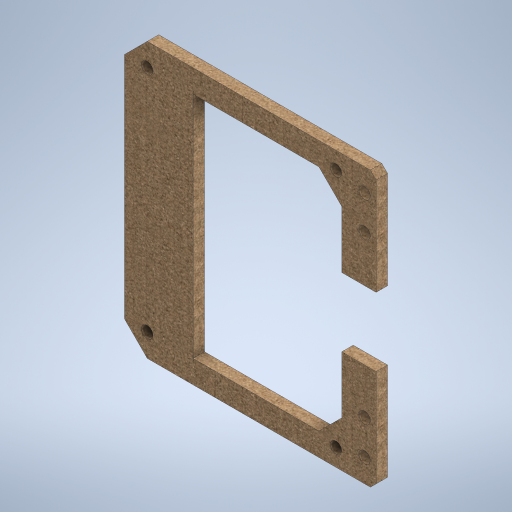
# Autodesk Inventor part: MarcoV2
Saved by Autodesk Inventor 2023.1 (Build 271208000, 208)
## iProperties
Created: 2022-10-30
Part Number: MarcoV2
Material: MDF Medium Density Fiberboard
Document SubType Name: Modeling
Designer: Daniel Peña
Density: 0.8 g/cm^3
Appearance: Cardboard - Corrugated
Author: Daniel Peña
Autodesk Inventor part; units mm, degrees
ref_plane "YZ Plane" through (0, 0, 0) normal (1, 0, 0) x (0, 1, 0)
ref_plane "XZ Plane" through (0, 0, 0) normal (0, 1, 0) x (-1, 0, 0)
ref_plane "XY Plane" through (0, 0, 0) normal (0, 0, 1) x (1, 0, 0)
sketch "Sketch1" plane through (0, 0, 0) normal (0, 0, 1) x (1, 0, 0)
  line L0 (-175, -7.5) -> (-230, -7.5)
  line L1 (-250, 2.5) -> (-152.5, 2.5)
  line L2 (-82.5, -57.5) -> (-255, -57.5)
  line L3 (-150, -42.5) -> (-165, -42.5)
  line L4 (-150, 0) -> (-150, -42.5)
  line L5 (-175, -7.5) -> (-165, -17.5)
  line L6 (-165, -42.5) -> (-165, -17.5)
  line L7 (-175, -107.5) -> (-230, -107.5)
  line L8 (-250, -117.5) -> (-152.5, -117.5)
  line L9 (-150, -72.5) -> (-165, -72.5)
  line L10 (-150, -115) -> (-150, -72.5)
  line L11 (-175, -107.5) -> (-165, -97.5)
  line L12 (-165, -72.5) -> (-165, -97.5)
  line L13 (-230, -7.5) -> (-230, -107.5)
  line L14 (-260, -107.5) -> (-260, -7.5)
  line L15 (-250, 2.5) -> (-260, -7.5)
  line L16 (-250, -117.5) -> (-260, -107.5)
  line L17 (-152.5, 2.5) -> (-150, 0)
  line L18 (-152.5, -117.5) -> (-150, -115)
  point P0 (0, 0)
  point P1 (-260, 2.5)
  point P2 (-152.5, 2.5)
  point P3 (-260, -117.5)
  point P4 (-150, 2.5)
  point P5 (-150, -117.5)
  dimension "d2" = -7.5
  dimension "d4" = 10
  dimension "d40" = 15
  dimension "d53" = 10
  dimension "d54" = 10
  dimension "d56" = 65
  dimension "d57" = 30
  dimension "d58" = 10
  dimension "d59" = 10
  dimension "d60" = 10
  dimension "d61" = 10
  dimension "d69" = 45
  dimension "d70" = 2.5
  dimension "d71" = 2.5
  dimension "d72" = 2.5
  dimension "d73" = 2.5
  constraints: 38 end point, 9 point on line, 6 symmetric about line, 3 vertical, 2 horizontal
  measures "d2" distance from line of L0 point (0, 0)
  measures "d4" distance between parallel lines of L0 L1
  measures "d40" distance between parallel lines of L4 L6
  measures "d53" horizontal distance of L0.start L5.end
  measures "d54" horizontal distance of L0.start L5.end
  measures "d56" distance between parallel lines of L13 L12
  measures "d57" distance between parallel lines of L14 L13
  measures "d58" distance of L1.start point (-260, 2.5)
  measures "d59" distance of L14.end point (-260, 2.5)
  measures "d60" distance of L8.start point (-260, -117.5)
  measures "d61" distance of L14.start point (-260, -117.5)
  measures "d69" distance of point (-150, 2.5) L3.start
  measures "d70" distance of L1.end point (-150, 2.5)
  measures "d71" distance of L4.start point (-150, 2.5)
  measures "d72" distance of L8.end point (-150, -117.5)
  measures "d73" distance of L10.start point (-150, -117.5)
extrude "Extrusion1" add sketch "Sketch1" along normal blind 5
sketch "Sketch3" plane through (0, 0, 5) normal (0, 0, 1) x (1, 0, 0)
  line L0 (-155, 3.7259) -> (-155, -113.632) construction
  line L1 (-150, -42.5) -> (-150, 0) construction
  line L2 (-225, -107.5) -> (-225, -7.5) construction
  line L3 (-225, -57.375) -> (-3.3098, -57.375) construction
  point P0 (0, 0)
  point P1 (-150, 5)
  point P2 (-155, -7.375)
  point P3 (-155, -22.375)
  point P4 (-155, -92.375)
  point P5 (-155, -107.375)
  point P6 (-230, -7.5)
  dimension "d41" = 5
  dimension "d42" = 15
  dimension "d43" = 70
  constraints: 4 end point, 4 point on line, 2 symmetric about line, 1 horizontal, 1 vertical, 2 other
  measures "d41" distance between parallel lines of L0 L1
  measures "d42" distance of point (-155, -92.375) point (-155, -107.375)
  measures "d43" distance of point (-155, -92.375) point (-155, -22.375)
hole "Hole2" at (-155, -7.375, 5) at (-155, -22.375, 5) at (-155, -92.375, 5) at (-155, -107.375, 5) direction (0, 0, -1) diameter 5 end through all
sketch "Sketch4" plane through (0, 0, 5) normal (0, 0, 1) x (1, 0, 0)
  circle A0 centre (-250, -7.5) radius 2.5 projected
  circle A1 centre (-250, -107.5) radius 2.5 projected
  circle A2 centre (-167.5, -5) radius 2.5 projected
  circle A3 centre (-167.5, -110) radius 2.5 projected
  point P0 (0, 0)
  constraints: 4 coincident
hole "Hole3" at (-167.5, -5, 5) at (-167.5, -110, 5) at (-250, -107.5, 5) at (-250, -7.5, 5) direction (0, 0, -1) diameter 5 end through all
equation "\"d59\" = d58"
equation "\"d60\" = d58"
equation "\"d61\" = d60"
equation "\"d71\" = d70"
equation "\"d72\" = d70"
equation "\"d73\" = d72"
body "Solid1"
